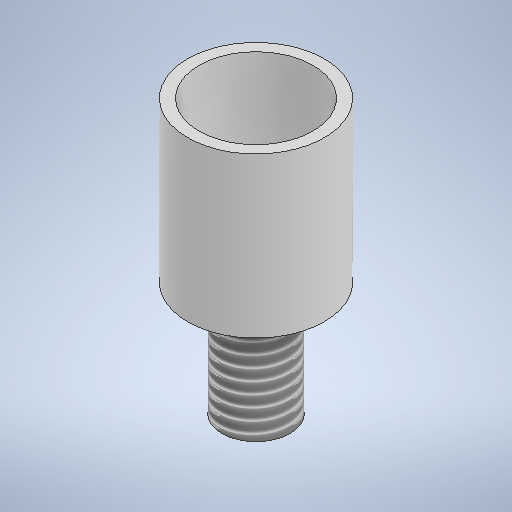
# Autodesk Inventor part: NozzleAttachment
Saved by Autodesk Inventor 2025.2 (Build 292293000, 293)
## iProperties
Created: 2025-05-29
Part Number: NozzleAttachment
Material: Generic
Document SubType Name: Modeling
Designer: Simon
Density: 1 g/cm^3
Appearance: Default
Author: Simon
Autodesk Inventor part; units mm, degrees
ref_plane "YZ Plane" through (0, 0, 0) normal (1, 0, 0) x (0, 1, 0)
ref_plane "XZ Plane" through (0, 0, 0) normal (0, 1, 0) x (-1, 0, 0)
ref_plane "XY Plane" through (0, 0, 0) normal (0, 0, 1) x (1, 0, 0)
sketch "Sketch1" plane through (0, 0, 0) normal (0, 1, 0) x (-1, 0, 0)
  circle A0 centre (0, 0) radius 3
  circle A1 centre (0, 0) radius 2.5
  dimension "d0" = 6
  dimension "d1" = 5
  constraints: 2 centre point, 2 coincident
  measures "d0" diameter of A0
  measures "d1" diameter of A1
extrude "Extrusion1" add sketch "Sketch1" along normal blind 6
sketch "Sketch2" plane through (0, 0, 0) normal (0, -1, 0) x (1, 0, 0)
  circle A0 centre (0, 0) radius 1
  circle A1 centre (0, 0) radius 3
  dimension "d6" = 2
  constraints: 2 centre point, 1 coincident
  measures "d6" diameter of A0
extrude "Extrusion2" add sketch "Sketch2" along normal blind 1
sketch "Sketch3" plane through (0, -1, 0) normal (0, -1, 0) x (1, 0, 0)
  circle A0 centre (0, 0) radius 1.5
  circle A1 centre (0, 0) radius 1
  dimension "d9" = 3
  constraints: 2 centre point, 2 coincident
  measures "d9" diameter of A0
extrude "Extrusion3" add sketch "Sketch3" along normal blind 5
thread "Thread2" size "M3x0.5" class "6g" standard "ISO Metric profile" full length
body "Solid1"
